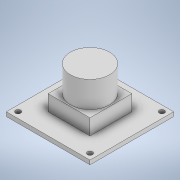
# Autodesk Inventor part: cam_1
Saved by Autodesk Inventor 2020 (Build 240168000, 168)
## iProperties
Created: 2020-05-02
Part Number: cam_1
Material: Generic
Document SubType Name: Modeling
Designer: psrobotics
Density: 1 g/cm^3
Appearance: Default
Author: psrobotics
Autodesk Inventor part; units mm, degrees
ref_plane "YZ Plane" through (0, 0, 0) normal (1, 0, 0) x (0, 1, 0)
ref_plane "XZ Plane" through (0, 0, 0) normal (0, 1, 0) x (-1, 0, 0)
ref_plane "XY Plane" through (0, 0, 0) normal (0, 0, 1) x (1, 0, 0)
sketch "Sketch1" plane through (0, 0, 0) normal (0, 1, 0) x (-1, 0, 0)
  line L0 (-16, 16) -> (-16, -16)
  line L1 (-16, -16) -> (16, -16)
  line L2 (16, -16) -> (16, 16)
  line L3 (16, 16) -> (-16, 16)
  line L4 (-16, 16) -> (16, -16) construction
  line L5 (-16, -16) -> (16, 16) construction
  point P0 (0, 0)
  dimension "d0" = 32
  dimension "d1" = 32
  constraints: 12 end point, 2 midpoint, 2 parallel, 1 perpendicular, 1 vertical
  measures "d0" distance of L0.start L0.end
  measures "d1" distance of L1.end L0.end
extrude "Extrusion1" add sketch "Sketch1" along normal blind 1.6
sketch "Sketch2" plane through (0, 1.6, 0) normal (0, 1, 0) x (1, 0, 0)
  line L0 (-8, -8) -> (-8, 8)
  line L1 (-8, 8) -> (8, 8)
  line L2 (8, 8) -> (8, -8)
  line L3 (8, -8) -> (-8, -8)
  line L4 (-8, -8) -> (8, 8) construction
  line L5 (-8, 8) -> (8, -8) construction
  point P0 (0, 0)
  dimension "d4" = 16
  dimension "d5" = 16
  constraints: 12 end point, 2 midpoint, 2 parallel, 1 perpendicular, 1 vertical
  measures "d4" distance of L0.start L0.end
  measures "d5" distance of L0.end L1.end
extrude "Extrusion2" add sketch "Sketch2" along normal blind 6
sketch "Sketch3" plane through (0, 7.6, 0) normal (0, 1, 0) x (1, 0, 0)
  circle A0 centre (0, 0) radius 7.5
  dimension "d8" = 15
  constraints: 1 centre point, 1 coincident
  measures "d8" diameter of A0
extrude "Extrusion3" add sketch "Sketch3" along normal blind 10
sketch "Sketch4" plane through (0, 1.6, 0) normal (0, 1, 0) x (1, 0, 0)
  line L0 (-13.75, -13.75) -> (-13.75, 13.75)
  line L1 (-13.75, 13.75) -> (13.75, 13.75)
  line L2 (13.75, 13.75) -> (13.75, -13.75)
  line L3 (13.75, -13.75) -> (-13.75, -13.75)
  line L4 (-13.75, -13.75) -> (13.75, 13.75) construction
  line L5 (-13.75, 13.75) -> (13.75, -13.75) construction
  point P0 (0, 0)
  dimension "d11" = 27.5
  dimension "d12" = 27.5
  constraints: 12 end point, 2 midpoint, 2 parallel, 1 perpendicular, 1 vertical
  measures "d11" distance of L0.start L0.end
  measures "d12" distance of L0.end L1.end
hole "Hole1" at (-13.75, 1.6, 13.75) at (13.75, 1.6, 13.75) at (13.75, 1.6, -13.75) at (-13.75, 1.6, -13.75) direction (0, -1, 0) diameter 2 depth 7
body "Solid1"
